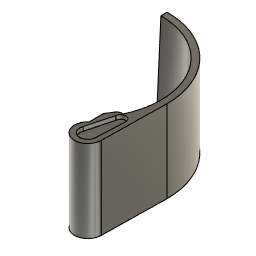
Pince droite principlae v3 (Autodesk Fusion 360 design; units mm, degrees)
Autodesk Fusion 360 part; units mm, degrees
sketch "Esquisse1" plane through (0, 0, 0) normal (0, 0, 1) x (1, 0, 0)
  circle A0 centre (103.6528, -35.0482) radius 2
  line L0 (105.3719, -17.8125) -> (108.4663, -31.4663)
  line L1 (104.2236, -27.2236) -> (96.5224, -27.2236)
  line L2 (108.4663, -17.4663) -> (105.9663, -17.4663)
  line L3 (108.4663, -31.4663) -> (104.9663, -31.4663)
  line L4 (108.4663, -17.4663) -> (106.4663, -17.4663)
  line L5 (108.4663, -17.4663) -> (110.9663, -17.4663)
  circle A1 centre (110.5862, -17.6277) radius 2.5
  circle A2 centre (108.4663, -17.4663) radius 2
  line L6 (108.4663, -31.4663) -> (95.6303, -41.0181)
  line L7 (104.5124, -30.8605) -> (108.1151, -17.2491)
  line L8 (108.4663, -31.4663) -> (108.4663, -15.4663)
  line L9 (114.9663, -31.4663) -> (115.5, 0)
  line L10 (108.4663, -31.4663) -> (104.5124, -30.8605)
  line L11 (0, 0) -> (0, -38.5)
  line L12 (77, 0) -> (77, 38.5)
  line L13 (77, -38.5) -> (108.4797, -38.5)
  line L14 (0, 0) -> (-27.2236, -27.2236)
  line L15 (43.5, 30) -> (33.5, 30)
  line L16 (77, 0) -> (38.5, 0)
  line L17 (108.4663, -31.4663) -> (108.4663, -38.5)
  line L18 (108.4663, -31.4663) -> (115.5, -19.3614)
  line L19 (108.4663, -31.4663) -> (111.9259, -31.9962)
  line L20 (109.6978, -23.0708) -> (113.709, -20.0859)
  line L21 (108.4663, -31.4663) -> (110.5862, -17.6277)
  line L22 (116.8617, -32.6978) -> (120.8729, -29.7129)
  line L23 (108.4663, -31.4663) -> (112.4201, -32.072)
  line L24 (112.4201, -32.072) -> (113.0574, -18.0063)
  line L25 (108.4663, -31.4663) -> (112.4663, -31.4663)
  line L26 (110.5862, -17.6277) -> (113.0574, -18.0063)
  line L27 (108.4663, -31.4663) -> (112.0482, -36.2797)
  line L28 (113.709, -20.0859) -> (120.8729, -29.7129)
  line L29 (115.5, -31.4663) -> (115.5, 0)
  line L30 (108.4663, -31.4663) -> (111.9663, -31.4663)
  line L31 (116.8617, -32.6978) -> (112.0482, -36.2797)
  line L32 (109.6978, -23.0708) -> (116.8617, -32.6978)
  line L33 (112.4663, -31.4663) -> (115.5, -31.4663)
  line L34 (109.9031, -21.6716) -> (118.2609, -32.9031)
  line L35 (108.4663, -17.4663) -> (110.4663, -17.4663)
  line L36 (110.9663, -17.4663) -> (112.4663, -31.4663)
  line L37 (110.5862, -17.6277) -> (108.1151, -17.2491)
  line L38 (110.4663, -17.4663) -> (111.9663, -31.4663)
  line L39 (0, 0) -> (-38.5, 0)
  line L40 (33.5, 30) -> (33.5, 0)
  line L41 (43.5, 0) -> (43.5, 30)
  circle A3 centre (0, 0) radius 33.5
  circle A4 centre (108.4663, -31.4663) radius 6
  line L42 (105.9663, -17.4663) -> (104.4663, -31.4663)
  circle A5 centre (108.4663, -31.4663) radius 4
  line L43 (104.8843, -26.6528) -> (109.6978, -23.0708)
  line L44 (95.6303, -41.0181) -> (92.0483, -36.2046)
  circle A6 centre (108.4663, -31.4663) radius 14
  line L45 (92.0483, -36.2046) -> (88.0371, -39.1895)
  circle A7 centre (108.4663, -31.4663) radius 7.0337
  line L46 (104.2236, -27.2236) -> (108.4663, -31.4663)
  line L47 (77, -38.5) -> (0, -38.5)
  line L48 (0, 0) -> (0, 38.5)
  line L49 (38.5, 50) -> (38.5, -50)
  line L50 (33.5, 0) -> (43.5, 0)
  circle A8 centre (77, 0) radius 38.5
  circle A9 centre (77, 0) radius 32.5
  line L51 (77, 0) -> (104.2236, -27.2236)
  line L52 (112.0482, -36.2797) -> (99.2122, -45.8316)
  line L53 (0, 0) -> (38.5, 0)
  circle A10 centre (0, 0) radius 38.5
  line L54 (99.007, -47.2308) -> (118.2609, -32.9031)
  circle A11 centre (103.6528, -35.0482) radius 2.5
  circle A12 centre (108.4663, -17.4663) radius 2.5
  line L55 (90.6491, -35.9993) -> (99.007, -47.2308)
  circle A13 centre (108.4663, -31.4663) radius 2.5
  circle A14 centre (108.4663, -31.4663) radius 6.5
  line L56 (88.0371, -39.1895) -> (95.201, -48.8165)
  line L57 (104.2236, -27.2236) -> (104.2236, -19.5224)
  line L58 (108.4663, -31.4663) -> (104.4663, -31.4663)
  line L59 (90.6491, -35.9993) -> (109.9031, -21.6716)
  circle A15 centre (108.4663, -31.4663) radius 3.5
  line L60 (99.2122, -45.8316) -> (95.6303, -41.0181)
  line L61 (106.4663, -17.4663) -> (104.9663, -31.4663)
  line L62 (104.8843, -26.6528) -> (92.0483, -36.2046)
  line L63 (108.4663, -31.4663) -> (104.8843, -26.6528)
  line L64 (99.2122, -45.8316) -> (95.201, -48.8165)
  circle A16 centre (77, 0) radius 33.5
  circle A17 centre (0, 0) radius 32.5
  line L65 (77, 0) -> (115.5, 0)
  line L66 (77, 0) -> (77, -38.5)
  dimension "d1" = 65
  dimension "d2" = 67
  dimension "d3" = 77
  dimension "d4" = 10
  dimension "d5" = 30
  dimension "d6" = 77
  dimension "d7" = 43.5
  dimension "d8" = 67
  dimension "d9" = 65
  dimension "d10" = 45
  dimension "d11" = 45
  dimension "d12" = 6
  dimension "d13" = 12
  dimension "d14" = 16
  dimension "d15" = 6
  dimension "d16" = 1
  dimension "d17" = 1
  dimension "d18" = 1
  dimension "d19" = 24
  dimension "d20" = 24
  dimension "d21" = 38.5
  dimension "d22" = 5
  dimension "d23" = 5
  dimension "d24" = 5
  dimension "d25" = 5
  dimension "d26" = 4
  dimension "d27" = 5
  dimension "d28" = 7
  dimension "d29" = 16
  dimension "d30" = 4
  dimension "d31" = 2
  dimension "d32" = 13
  dimension "d33" = 5
  dimension "d34" = 5
  dimension "d35" = 8
  dimension "d36" = 100
  dimension "d37" = 5
  dimension "d38" = 20
  dimension "d39" = 21.45
  dimension "d40" = 5
  dimension "d41" = 31.4663
  dimension "d42" = 45
  dimension "d43" = 45
  constraint coincident L11.start L14.start
  constraint concentric A3 A17
  constraint coincident L16.end A10
  constraint horizontal L53
  constraint horizontal L50
  constraint vertical L41
  constraint horizontal L15
  constraint vertical L40
  constraint coincident L40.end A3
  constraint coincident L40.end L53
  constraint coincident L11.end A10
  constraint vertical L11
  constraint concentric A8 A16
  constraint concentric A8 A9
  constraint coincident L12.start L16.start
  constraint parallel L16 L53
  constraint coincident L13.start A8
  constraint perpendicular L16 L66
  constraint coincident L9.end A8
  constraint horizontal L65
  constraint coincident L1.start A8
  constraint coincident L39.end A10
  constraint horizontal L39
  constraint coincident L14.end A10
  constraint parallel L46 L51
  constraint coincident L0.end L3.start
  constraint coincident L43.start A4
  constraint perpendicular L6 L63
  constraint perpendicular L62 L63
  constraint coincident L27.end A4
  constraint perpendicular L6 L27
  constraint tangent A4 L52
  constraint perpendicular L52 L60
  constraint tangent A4 L43
  constraint perpendicular L32 L62
  constraint perpendicular L31 L32
  constraint perpendicular L44 L62
  constraint parallel L55 L60
  constraint perpendicular L54 L55
  constraint perpendicular L55 L59
  constraint perpendicular L45 L55
  constraint perpendicular L55 L64
  constraint perpendicular L20 L34
  constraint perpendicular L22 L32
  constraint coincident L48.end A10
  constraint vertical L48
  constraint coincident L12.end A8
  constraint parallel L12 L48
  constraint coincident A0.centre A4
  constraint coincident A0.centre L6
  constraint concentric A4 A13
  constraint concentric A13 A15
  constraint vertical L8
  constraint coincident L2.start L8
  constraint coincident L2.start L4.start
  constraint coincident L35.end A2
  constraint perpendicular L8 L35
  constraint coincident L4.end A2
  constraint perpendicular L4 L8
  constraint coincident L3.end A15
  constraint horizontal L3
  constraint coincident L30.end A15
  constraint horizontal L30
  constraint concentric A14 A15
  constraint concentric A0 A11
  constraint concentric A2 A12
  constraint coincident L42.end A5
  constraint parallel L3 L58
  constraint coincident L25.end A5
  constraint horizontal L25
  constraint coincident L2.end A12
  constraint perpendicular L2 L8
  constraint coincident L5.end A12
  constraint parallel L2 L5
  constraint perpendicular L47 L49
  constraint perpendicular L13 L66
  constraint concentric A5 A7
  constraint tangent L13 A7
  constraint coincident L17.end A7
  constraint perpendicular L13 L17
  constraint concentric A6 A14
  constraint coincident L2.start A6
  constraint coincident L29.start A7
  constraint horizontal L33
  constraint perpendicular L29 L65
  constraint coincident L0.start A16
  constraint coincident L0.start A6
  constraint coincident L18.end L29
  constraint coincident L18.end A6
  constraint coincident A1.centre A6
  constraint coincident A1.centre L21.end
  constraint coincident L7.end A1
  constraint perpendicular L21 L37
  constraint coincident L24.end A1
  constraint perpendicular L21 L26
  constraint coincident L7.start A5
  constraint perpendicular L10 L21
  constraint coincident L19.end A15
  constraint perpendicular L19 L21
  constraint coincident L23.end A5
  constraint parallel L19 L23
  constraint coincident L9.start L33
  constraint coincident L9.start A14
  constraint coincident L1.end A16
  constraint coincident L57.end A16
  measures "d1" diameter of A17
  measures "d2" diameter of A3
  measures "d3" diameter of A10
  measures "d4" distance of L41.start L40.end
  measures "d5" distance of L15.start L41.start
  measures "d6" diameter of A8
  measures "d7" distance of L12.start L40
  measures "d8" diameter of A16
  measures "d9" diameter of A9
  measures "d10" angle of L51 L65
  measures "d11" angle of L14 L39
  measures "d12" distance of L1.start L0.end
  measures "d13" diameter of A4
  measures "d14" distance of L6.end L0.end
  measures "d15" distance of L0.end L32
  measures "d16" distance of L55 L60
  measures "d17" distance of L52 L54
  measures "d18" distance of L59 L62
  measures "d19" distance of L34.end L54.start
  measures "d20" distance of L34.start L55.start
  measures "d21" distance of L12.start L55.start
  measures "d22" distance of L44.end L45.end
  measures "d23" distance of L56.end L52.end
  measures "d24" distance of L20.start L20.end
  measures "d25" distance of L22.start L22.end
  measures "d26" diameter of A0
  measures "d27" diameter of A13
  measures "d28" diameter of A15
  measures "d29" distance of L0.end L8.end
  measures "d30" diameter of A2
  measures "d31" distance of L2.start L8.end
  measures "d32" diameter of A14
  measures "d33" diameter of A11
  measures "d34" diameter of A12
  measures "d35" diameter of A5
  measures "d36" distance of L49.start L49.end
  measures "d37" distance of L41 L49
  measures "d38" distance of L49.start L15
  measures "d39" angle of L18 L21
  measures "d40" diameter of A1
  measures "d41" vertical distance of L9.end L9.start
  measures "d42" angle of L1 L51
  measures "d43" angle of L51 L57
extrude "Extrusion1" add sketch "Esquisse1" along normal blind 40 contours A0 L6 A4 | A0 A4 A5 A11 | A0 L6 A4 | L6 A5 A11 | A0 A4 A5 A11 | L6 A5 A11 | A0 A4 A11 A14 | A0 L6 A4 A14 | A0 L6 A4 A14 | A0 A4 A11 A14 | L3 L6 A13 L58 A15 | L17 A5 A11 A15 | A5 A11 L58 A15 | L6 L17 A13 A15 | A4 L42 A5 L46 A11 | L17 A4 A5 A11 | L17 A4 A11 A14 | A4 A8 A11 A14 | L3 L6 A13 L58 | L6 L17 A13 | L3 L10 A13 L58 L61 | L10 L42 L58 A15 | L10 A15 L61 | L17 L27 A5 A15 | L17 L27 A13 A15 | L10 L42 A5 | L17 L27 A4 A5 | L17 A4 L52 A14 | L1 A8 A14 L62 | A4 A8 L62 | A4 L42 L46 L63 | A8 L57 L62 | L1 L51 L62 | L51 L57 L62 | L0 A13 L63 | L0 L8 A13 | L3 L10 A13 L58 | L17 L27 A13 | L18 L21 A13 | L19 L23 L25 L30 A13 | L8 L21 A13 | L18 L25 L30 A13 | L19 L23 L27 A13 | L10 L46 A13 | L46 A13 L63 | L10 A15 L61 | L7 L10 L42 A5 A15 L61 | L10 L46 A13 A15 L61 | L23 L27 A5 A15 | L19 L23 L27 A13 A15 | L7 L10 L42 | L7 L42 A5 | L27 L33 A4 A5 | L31 L33 A4 A14 | L31 L52 A14 | L1 A14 L62 | L1 L51 A14 L62 | A4 L42 L43 A8 L62 | A4 L42 L43 L63 | L7 L42 A5 L46 | L7 L42 L46 L61 L63 | L42 A8 A14 L57 L62 | L51 A14 L57 L62 | L0 A13 A15 L63 | L0 L8 A13 A15 | L8 L21 A13 A15 | L18 L21 A13 A15 | L18 L25 L30 L38 A13 A15 | L19 L23 L25 L30 A13 A15 | L46 A13 A15 L63 | A5 L46 A15 L61 | L23 L24 L25 A15 | L7 L42 A5 | L24 L25 A5 | L32 L33 A4 A14 | L24 L33 A4 A5 | A4 L43 L61 | A4 L42 L61 L63 | L42 L43 A8 L61 | L7 A5 L46 L61 | L7 L46 L61 | L42 A8 A14 L61 | L42 A7 A14 L57 L59 | L0 A5 A15 L63 | L0 L8 A5 A15 | L8 L21 A5 A15 | L18 L21 A5 A15 | L18 L38 A5 A15 | L24 L25 L36 L38 A5 A15 | L38 A15 | A5 L46 A15 L63 | A5 L46 L61 | L24 L25 L36 | L24 L36 A5 | L9 L32 A14 | L24 L32 A4 | L24 L32 A14 | L7 A4 L43 L61 | L7 A4 L61 L63 | L7 L43 A8 A14 L61 | L7 L61 L63 | L7 A5 L46 L61 L63 | L42 A7 A14 L61 | A8 A14 L61 | A7 L57 L59 | L0 L7 A4 A5 L63 | L0 L8 A4 A5 | L8 L21 A4 A5 | L18 L21 L38 A4 A5 | L18 L38 A5 | L24 L36 A5 | L24 L36 A4 A5 | L9 L24 L32 L34 A7 A14 | L24 L32 L36 A14 | L24 L32 L36 A4 | L0 L7 A4 L43 A14 | L7 L43 A14 | L42 A7 L59 | L42 A7 L59 L61 | L7 A7 A8 A14 L61 | L7 A8 A14 | L0 L42 A7 L57 L59 A16 | L0 L8 A4 A14 | L8 L21 A4 A14 | L18 L38 A4 | L18 L36 L38 A4 A5 | L21 L38 A4 A14 | L9 L34 A7 | L18 L24 L36 A7 A14 | L18 L32 L36 A4 A14 | L32 L36 A14 | L0 L7 L43 A7 A8 A14 | L0 L43 A14 | L0 L42 L59 L61 | L7 A7 L59 L61 | L7 A7 A8 | L0 L8 L43 A7 A14 | L8 L21 A7 A14 | L18 L38 A4 A14 | L21 L32 L38 A7 A14 | L9 L18 L24 L28 L34 A7 | L34 A7 | L18 L24 L34 A7 | L24 L34 A7 | L18 L32 L36 A14 | L18 L32 A14 | L0 L43 A7 | L0 L42 A6 A12 L61 | L0 L42 A6 | L0 L7 L59 L61 | L0 L7 A7 A8 L59 | L0 A7 A8 | L42 A6 A12 A16 | L8 L43 A7 | L8 L21 L32 L43 A7 | L18 L32 L38 A14 | L21 L32 A7 | L9 L18 L28 | L18 L24 L34 | L18 L34 L36 A7 | L18 L36 A7 | L18 L32 L36 L38 A7 | L0 L8 L43 A7 A8 L59 | L0 L7 A12 L61 | L42 A6 A12 | L0 L7 L59 | L0 A8 L59 | L2 A1 A2 A12 A16 | A12 A16 | L8 L20 L21 L34 L43 L59 | L32 L38 A7 | L20 L21 L32 | L20 L21 L32 L34 L38 A7 | L9 L18 L20 L24 L28 A6 | L12 A8 A16 L65 | A1 L9 A8 A12 A16 L65 | A1 L9 L24 A6 A8 | L18 L20 L24 L28 | L18 L20 L24 L34 L36 | L34 L36 L38 A7 | L0 L7 L8 A8 A12 L59 | A2 L7 A6 A12 L61 | A6 A12 L61 | L2 A6 A12 L61 | L8 A8 L59 | A1 L8 L21 L34 A8 L59 | L20 L21 L34 | A1 L24 A6 | A1 L20 L24 L36 A6 | L20 L34 L36 L38 | A2 L7 L8 A12 | A2 A6 L61 | L2 L4 A1 A2 L7 L8 | L2 L4 A2 L7 A6 | A1 L8 A8 A12 | L5 A1 A2 A12 | A1 L26 L36 A8 A12 | L20 L34 L38 | A1 L20 L21 L34 L38 | A1 L26 A8 | A1 L26 A6 A8 | A1 L36 A6 A8 | A1 L20 L36 L38 | A1 A2 L7 L8 A6 | A2 L7 A6 | A1 A2 L8 A12 | L2 L4 A1 L7 | L2 L4 A1 L7 A6 | A1 A2 L8 | A1 L21 A8 | A1 L21 A8 A12 | L5 A1 A2 L8 L35 L37 | L5 L26 L37 L38 A6 A12 | L26 L36 A12 | A1 L21 L38 A8 | L26 L36 A6 A8 | A1 L36 L38 A8 | L36 A6 A8 | A1 A2 L8 | A1 A2 L21 L37 L38 A6 A12 | L2 L4 A1 L8 L37 | L2 L4 A1 A6 | A1 L8 L37 | L21 L38 A8 A12 | L5 A2 L35 L37 | A2 L37 L38 A6 | L26 L36 A6 A12 | L26 A6 A12 | L36 L38 A6 A8 A12 | A1 A2 L8 A6 | A1 L8 A6 | L21 L38 A12 | L5 L8 L35 L37 | L5 L35 L37 A6 | L21 L37 L38 A6 | L21 L38 A6 A12 picked at (104.2904, -25.8214)
chamfer "Chanfrein1" distance 2 distance2 40 1 edges at (105.8116, 17.0921, 40) measured on face at (108.9471, -32.5187, 40)
sketch "Esquisse2" plane through (0, 0, 40) normal (0, 0, 1) x (-1, 0, 0)
  arc A0 (-109.1469, 15.0607) -> (-77, -35.5) centre (-77, 0) ccw
  arc A1 (-109.1469, 15.0607) -> (-106.1789, 16.4572) centre (-108.4663, 17.4663) ccw
  arc A2 (-104.2236, 19.5224) -> (-106.1789, 16.4572) centre (-77, 0) ccw
  line L0 (-104.2236, 19.5224) -> (-104.2236, 26.5418)
  arc A3 (-104.2236, 26.5418) -> (-114.9663, 31.4663) centre (-108.4663, 31.4663) ccw
  line L1 (-114.9663, 31.4663) -> (-115.5, 0)
  arc A4 (-115.5, 0) -> (-77, -38.5) centre (-77, 0) ccw
  line L2 (-77, -38.5) -> (-77, -35.5)
  circle A5 centre (-103.6528, 35.0482) radius 2
  line L3 (-105.3719, 17.8125) -> (-108.4663, 31.4663)
  line L4 (-104.2236, 27.2236) -> (-96.5224, 27.2236)
  line L5 (-108.4663, 17.4663) -> (-105.9663, 17.4663)
  line L6 (-108.4663, 31.4663) -> (-104.9663, 31.4663)
  line L7 (-108.4663, 17.4663) -> (-106.4663, 17.4663)
  line L8 (-108.4663, 17.4663) -> (-110.9663, 17.4663)
  circle A6 centre (-110.5862, 17.6277) radius 2.5
  circle A7 centre (-108.4663, 17.4663) radius 2
  line L9 (-108.4663, 31.4663) -> (-95.6303, 41.0181)
  line L10 (-104.5124, 30.8605) -> (-108.1151, 17.2491)
  line L11 (-108.4663, 31.4663) -> (-108.4663, 15.4663)
  line L12 (-114.9663, 31.4663) -> (-115.5, 0)
  line L13 (-108.4663, 31.4663) -> (-104.5124, 30.8605)
  line L14 (0, 0) -> (0, 38.5)
  line L15 (-77, 0) -> (-77, -38.5)
  line L16 (-77, 38.5) -> (-108.4797, 38.5)
  line L17 (0, 0) -> (27.2236, 27.2236)
  line L18 (-43.5, -30) -> (-33.5, -30)
  line L19 (-77, 0) -> (-38.5, 0)
  line L20 (-108.4663, 31.4663) -> (-108.4663, 38.5)
  line L21 (-108.4663, 31.4663) -> (-115.5, 19.3614)
  line L22 (-108.4663, 31.4663) -> (-111.9259, 31.9962)
  line L23 (-109.6978, 23.0708) -> (-113.709, 20.0859)
  line L24 (-108.4663, 31.4663) -> (-110.5862, 17.6277)
  line L25 (-116.8617, 32.6978) -> (-120.8729, 29.7129)
  line L26 (-108.4663, 31.4663) -> (-112.4201, 32.072)
  line L27 (-112.4201, 32.072) -> (-113.0574, 18.0063)
  line L28 (-108.4663, 31.4663) -> (-112.4663, 31.4663)
  line L29 (-110.5862, 17.6277) -> (-113.0574, 18.0063)
  line L30 (-108.4663, 31.4663) -> (-112.0482, 36.2797)
  line L31 (-113.709, 20.0859) -> (-120.8729, 29.7129)
  line L32 (-115.5, 31.4663) -> (-115.5, 0)
  line L33 (-108.4663, 31.4663) -> (-111.9663, 31.4663)
  line L34 (-116.8617, 32.6978) -> (-112.0482, 36.2797)
  line L35 (-109.6978, 23.0708) -> (-116.8617, 32.6978)
  line L36 (-112.4663, 31.4663) -> (-115.5, 31.4663)
  line L37 (-109.9031, 21.6716) -> (-118.2609, 32.9031)
  line L38 (-108.4663, 17.4663) -> (-110.4663, 17.4663)
  line L39 (-110.9663, 17.4663) -> (-112.4663, 31.4663)
  line L40 (-110.5862, 17.6277) -> (-108.1151, 17.2491)
  line L41 (-110.4663, 17.4663) -> (-111.9663, 31.4663)
  line L42 (0, 0) -> (38.5, 0)
  line L43 (-33.5, -30) -> (-33.5, 0)
  line L44 (-43.5, 0) -> (-43.5, -30)
  circle A8 centre (0, 0) radius 33.5
  circle A9 centre (-108.4663, 31.4663) radius 6
  line L45 (-105.9663, 17.4663) -> (-104.4663, 31.4663)
  circle A10 centre (-108.4663, 31.4663) radius 4
  line L46 (-104.8843, 26.6528) -> (-109.6978, 23.0708)
  line L47 (-95.6303, 41.0181) -> (-92.0483, 36.2046)
  circle A11 centre (-108.4663, 31.4663) radius 14
  line L48 (-92.0483, 36.2046) -> (-88.0371, 39.1895)
  circle A12 centre (-108.4663, 31.4663) radius 7.0337
  line L49 (-104.2236, 27.2236) -> (-108.4663, 31.4663)
  line L50 (-77, 38.5) -> (0, 38.5)
  line L51 (0, 0) -> (0, -38.5)
  line L52 (-38.5, -50) -> (-38.5, 50)
  line L53 (-33.5, 0) -> (-43.5, 0)
  circle A13 centre (-77, 0) radius 38.5
  circle A14 centre (-77, 0) radius 32.5
  line L54 (-77, 0) -> (-104.2236, 27.2236)
  line L55 (-112.0482, 36.2797) -> (-99.2122, 45.8316)
  line L56 (0, 0) -> (-38.5, 0)
  circle A15 centre (0, 0) radius 38.5
  line L57 (-99.0069, 47.2308) -> (-118.2609, 32.9031)
  circle A16 centre (-103.6528, 35.0482) radius 2.5
  circle A17 centre (-108.4663, 17.4663) radius 2.5
  line L58 (-90.6491, 35.9993) -> (-99.0069, 47.2308)
  circle A18 centre (-108.4663, 31.4663) radius 2.5
  circle A19 centre (-108.4663, 31.4663) radius 6.5
  line L59 (-88.0371, 39.1895) -> (-95.201, 48.8165)
  line L60 (-104.2236, 27.2236) -> (-104.2236, 19.5224)
  line L61 (-108.4663, 31.4663) -> (-104.4663, 31.4663)
  line L62 (-90.6491, 35.9993) -> (-109.9031, 21.6716)
  circle A20 centre (-108.4663, 31.4663) radius 3.5
  line L63 (-99.2122, 45.8316) -> (-95.6303, 41.0181)
  line L64 (-106.4663, 17.4663) -> (-104.9663, 31.4663)
  line L65 (-104.8843, 26.6528) -> (-92.0483, 36.2046)
  line L66 (-108.4663, 31.4663) -> (-104.8843, 26.6528)
  line L67 (-99.2122, 45.8316) -> (-95.201, 48.8165)
  circle A21 centre (-77, 0) radius 33.5
  circle A22 centre (0, 0) radius 32.5
  line L68 (-77, 0) -> (-115.5, 0)
  line L69 (-77, 0) -> (-77, 38.5)
  point P0 (0, 0)
  dimension "d48" = 65
  dimension "d49" = 67
  dimension "d50" = 77
  dimension "d51" = 10
  dimension "d52" = 30
  dimension "d53" = 77
  dimension "d54" = 43.5
  dimension "d55" = 67
  dimension "d56" = 65
  dimension "d57" = 45
  dimension "d58" = 45
  dimension "d59" = 6
  dimension "d60" = 12
  dimension "d61" = 16
  dimension "d62" = 6
  dimension "d63" = 1
  dimension "d64" = 1
  dimension "d65" = 1
  dimension "d66" = 24
  dimension "d67" = 24
  dimension "d68" = 38.5
  dimension "d69" = 5
  dimension "d70" = 5
  dimension "d71" = 5
  dimension "d72" = 5
  dimension "d73" = 4
  dimension "d74" = 5
  dimension "d75" = 7
  dimension "d76" = 16
  dimension "d77" = 4
  dimension "d78" = 2
  dimension "d79" = 13
  dimension "d80" = 5
  dimension "d81" = 5
  dimension "d82" = 8
  dimension "d83" = 100
  dimension "d84" = 5
  dimension "d85" = 20
  dimension "d86" = 21.45
  dimension "d87" = 5
  dimension "d89" = 45
  dimension "d90" = 45
  constraint coincident P0 L14.start
  constraint concentric A8 A22
  constraint coincident L19.end A15
  constraint coincident L43.end A8
  constraint coincident L43.end L56
  constraint coincident L14.end A15
  constraint concentric A13 A21
  constraint concentric A13 A14
  constraint coincident A0.centre A2.centre
  constraint parallel L19 L56
  constraint coincident L16.start A13
  constraint perpendicular L19 L69
  constraint coincident L1.end A13
  constraint coincident L4.start A13
  constraint coincident L42.end A15
  constraint coincident L17.end A15
  constraint parallel L49 L54
  constraint coincident A3.centre L3.end
  constraint coincident L46.start A9
  constraint perpendicular L9 L66
  constraint perpendicular L65 L66
  constraint coincident L30.end A9
  constraint perpendicular L9 L30
  constraint tangent A9 L55
  constraint perpendicular L55 L63
  constraint tangent A9 L46
  constraint perpendicular L35 L65
  constraint perpendicular L34 L35
  constraint perpendicular L47 L65
  constraint parallel L58 L63
  constraint perpendicular L57 L58
  constraint perpendicular L58 L62
  constraint perpendicular L48 L58
  constraint perpendicular L58 L67
  constraint perpendicular L23 L37
  constraint perpendicular L25 L35
  constraint coincident L51.end A15
  constraint coincident A4.end A13
  constraint parallel L15 L51
  constraint coincident A5.centre A9
  constraint coincident A5.centre L9
  constraint concentric A9 A18
  constraint concentric A18 A20
  constraint coincident A1.centre L11
  constraint coincident A1.centre L5.start
  constraint coincident L38.end A7
  constraint perpendicular L11 L38
  constraint coincident L7.end A7
  constraint perpendicular L7 L11
  constraint coincident L6.end A20
  constraint coincident L33.end A20
  constraint concentric A19 A20
  constraint concentric A5 A16
  constraint concentric A7 A17
  constraint coincident L45.end A10
  constraint parallel L6 L61
  constraint coincident L28.end A10
  constraint coincident L5.end A17
  constraint perpendicular L5 L11
  constraint coincident L8.end A17
  constraint parallel L5 L8
  constraint perpendicular L50 L52
  constraint perpendicular L16 L69
  constraint concentric A10 A12
  constraint tangent L16 A12
  constraint coincident L20.end A12
  constraint perpendicular L16 L20
  constraint concentric A11 A19
  constraint coincident A1.centre A11
  constraint coincident L32.start A12
  constraint perpendicular L32 L68
  constraint coincident L3.start A21
  constraint coincident L3.start A11
  constraint coincident L21.end L32
  constraint coincident L21.end A11
  constraint coincident A6.centre A11
  constraint coincident A6.centre L24.end
  constraint coincident L10.end A6
  constraint perpendicular L24 L40
  constraint coincident L27.end A6
  constraint perpendicular L24 L29
  constraint coincident L10.start A10
  constraint perpendicular L13 L24
  constraint coincident L22.end A20
  constraint perpendicular L22 L24
  constraint coincident L26.end A10
  constraint parallel L22 L26
  constraint coincident A3.end L36
  constraint coincident A3.end A19
  constraint coincident L4.end A21
  constraint coincident A2.start A21
  measures "d48" diameter of A22
  measures "d49" diameter of A8
  measures "d50" diameter of A15
  measures "d51" distance of L44.start L43.end
  measures "d52" distance of L18.start L44.start
  measures "d53" diameter of A13
  measures "d54" distance of A0.centre L43
  measures "d55" diameter of A21
  measures "d56" diameter of A14
  measures "d57" angle of L54 L68
  measures "d58" angle of L17 L42
  measures "d59" distance of L4.start A3.centre
  measures "d60" diameter of A9
  measures "d61" distance of L9.end A3.centre
  measures "d62" distance of A3.centre L35
  measures "d63" distance of L58 L63
  measures "d64" distance of L55 L57
  measures "d65" distance of L62 L65
  measures "d66" distance of L37.end L57.start
  measures "d67" distance of L37.start L58.start
  measures "d68" distance of A0.centre L58.start
  measures "d69" distance of L47.end L48.end
  measures "d70" distance of L59.end L55.end
  measures "d71" distance of L23.start L23.end
  measures "d72" distance of L25.start L25.end
  measures "d73" diameter of A5
  measures "d74" diameter of A18
  measures "d75" diameter of A20
  measures "d76" distance of A3.centre L11.end
  measures "d77" diameter of A7
  measures "d78" distance of A1.centre L11.end
  measures "d79" diameter of A19
  measures "d80" diameter of A16
  measures "d81" diameter of A17
  measures "d82" diameter of A10
  measures "d83" distance of L52.start L52.end
  measures "d84" distance of L44 L52
  measures "d85" distance of L52.start L18
  measures "d86" angle of L21 L24
  measures "d87" diameter of A6
  measures "d89" angle of L4 L54
  measures "d90" angle of L54 L60
extrude "Extrusion2" cut sketch "Esquisse2" against normal blind 2 contours L8 A6 A7 A17 | A6 L29 L39 A13 A17 | A6 L29 A13 | L8 A6 A7 L11 L38 L40 | L8 L29 L40 L41 A11 A17 | L29 L39 A17 | A6 L29 A11 A13 | L29 L39 A11 A13 | A6 L11 L40 | L8 A7 L38 L40 | A7 L40 L41 A11 | L29 L39 A11 A17 | L29 A11 A17 | A6 L23 L27 L39 A11 | A6 L39 A11 A13 | L39 A11 A13 | L5 L7 A6 L11 L40 | L8 L11 L38 L40 | L8 L38 L40 A11 | A6 A7 L24 L40 L41 A11 A17 | A6 A7 L11 A11 | L24 L40 L41 A11 | L39 L41 A11 A13 A17 | L24 L41 A11 A17 | A6 L23 L39 L41 | A6 L39 L41 A13 | L21 L23 L27 L37 L39 | L5 L7 A6 A11 | A6 L11 A11 | A6 A7 L11 | A6 A7 L11 A17 | L24 L41 A17 | L24 L41 A13 A17 | L21 L27 L37 | L3 L10 L11 A13 A17 L62 | L3 L10 L62 | A6 A7 L10 L11 A11 | A7 L10 L11 A17 | A6 L23 L24 L37 L41 | A6 L24 L41 A13 | L23 L37 L39 L41 | A6 L24 A13 A17 | A6 L11 A13 A17 | L21 L27 L37 A12 | L21 L37 L39 A12 | L3 A13 L62 | L3 L10 A12 A13 L62 | A6 L11 L24 L37 A13 L62 | A6 L24 A13 | L23 L37 L41 | L37 L39 L41 A12 | L21 L27 L39 A12 A19 | L21 L39 A12 | L3 L11 L46 A12 A13 L62 | L3 A12 A13 | L11 A13 L62 | L10 A12 A13 | L23 L24 L37 | L11 L23 L24 L37 L46 L62 | L23 L24 L35 L37 L41 A12 | L21 L35 L39 L41 A12 | L21 L35 L39 A19 | L27 L35 L39 A19 | L20 L30 A10 A20 | L26 L30 A10 A20 | L3 L46 A12 | L3 L10 L46 A12 A13 A19 | L23 L24 L35 | L35 L41 A12 | L21 L35 A19 | L21 L35 L41 A19 | L35 L39 A19 | L27 L35 L39 A9 | L27 L28 A10 | L27 L28 L39 | L27 L39 A10 | L20 A10 A16 A20 | L20 L30 A18 A20 | L22 L26 L30 A18 A20 | L26 L27 L28 A20 | L3 L11 L46 A12 A19 | L3 L46 A19 | L11 L46 A12 | L11 L24 L35 L46 A12 | L10 L46 A19 | L24 L35 A12 | L24 L35 L41 A12 A19 | L27 L39 A9 A10 | L21 L35 L39 A9 A19 | L21 L41 A9 A19 | L27 L28 L39 L41 A10 A20 | L27 L39 A10 | L9 A10 A16 | L9 L20 A18 A20 | L20 L30 A18 | L22 L26 L30 A18 | L22 L26 L28 L33 A18 A20 | L10 L45 A10 | L10 L45 A10 | L10 A10 L49 L64 | L10 L49 L64 | L3 L11 A9 A19 | L3 L10 A9 L46 A19 | L11 L24 A12 A19 | L3 L10 A9 A10 L66 | L24 L41 A9 A19 | L21 L39 L41 A9 A10 | L21 L41 A9 | L21 L28 L33 L41 A18 A20 | L41 A20 | L9 A10 A16 | L6 L9 A18 L61 A20 | A10 A16 L61 A20 | L9 L20 A18 | L3 A18 L66 | L6 L9 A18 L61 | L3 L11 A18 | L6 L13 A18 L61 | L21 L24 A18 | L22 L26 L28 L33 A18 | L11 L24 A18 | L21 L28 L33 A18 | L13 L49 A18 | L49 A18 L66 | L10 L13 L45 | L10 L13 L45 A10 A20 L64 | L13 L45 A10 | L10 A10 L49 L64 L66 | A10 L49 L64 | L3 L11 A9 A10 | L11 L24 A9 A19 | L21 L24 L41 A9 A10 | L21 L41 A10 | L21 L41 A10 A20 | L6 L13 A18 L61 L64 | L13 L45 L61 A20 | L13 A20 L64 | L3 A18 A20 L66 | L3 L11 A18 A20 | L11 L24 A18 A20 | L13 L49 A18 A20 L64 | L21 L24 A18 A20 | L49 A18 A20 L66 | A10 L49 A20 L64 | A10 L49 A20 L66 | L3 L11 A10 A20 | L3 A10 A20 L66 | L11 L24 A9 A10 | L21 L24 A10 A20 | L13 A20 L64 | L11 L24 A10 A20 picked at (-108.5048, 19.1802)
sketch "Esquisse3" plane through (0, 0, 0) normal (0, 0, -1) x (1, 0, 0)
  arc A0 (114.9663, 31.4663) -> (104.2236, 26.5418) centre (108.4663, 31.4663) ccw
  line L0 (104.2236, 26.5418) -> (104.2236, 19.5224)
  arc A1 (106.1789, 16.4572) -> (104.2236, 19.5224) centre (77, 0) ccw
  arc A2 (106.1789, 16.4572) -> (106.4001, 16.0587) centre (108.4663, 17.4663) ccw
  arc A3 (77, -33.5) -> (106.4001, 16.0587) centre (77, 0) ccw
  line L1 (77, -33.5) -> (77, -38.5)
  arc A4 (77, -38.5) -> (115.5, 0) centre (77, 0) ccw
  line L2 (115.5, 0) -> (114.9663, 31.4663)
  circle A5 centre (108.4663, 31.4663) radius 6.5
  circle A6 centre (108.4663, 31.4663) radius 3
  dimension "d93" = 13
  dimension "d94" = 6
  constraint concentric A0 A5
  constraint concentric A5 A6
  measures "d93" diameter of A5
  measures "d94" diameter of A6
extrude "Extrusion3" cut sketch "Esquisse3" against normal blind 4 contours A6
